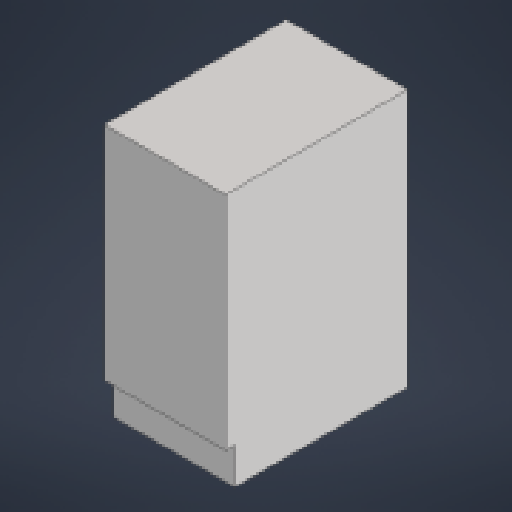
# Autodesk Inventor part: Mobile 40
Saved by Autodesk Inventor 2024.2 (Build 282272000, 272)
## iProperties
Created: 2025-08-13
Part Number: Mobile 40
Material: Generic
Document SubType Name: Modeling
Designer: Luca
Density: 1 g/cm^3
Appearance: Default
Author: Luca
Autodesk Inventor part; units mm, degrees
ref_plane "YZ Plane" through (0, 0, 0) normal (1, 0, 0) x (0, 1, 0)
ref_plane "XZ Plane" through (0, 0, 0) normal (0, 1, 0) x (-1, 0, 0)
ref_plane "XY Plane" through (0, 0, 0) normal (0, 0, 1) x (1, 0, 0)
sketch "Sketch1" plane through (0, 0, 0) normal (0, 1, 0) x (1, 0, 0)
  line L0 (200, 0) -> (-200, 0)
  line L1 (-200, 0) -> (-200, -600)
  line L2 (-200, -600) -> (200, -600)
  line L3 (200, -600) -> (200, 0)
  point P0 (0, 0)
  point P1 (0, 0)
  dimension "d0" = 400
  dimension "d1" = 600
  constraints: 8 end point, 2 parallel, 1 coincident, 1 horizontal, 1 midpoint, 1 perpendicular
  measures "d0" distance of L1.end L2.end
  measures "d1" distance of L0.end L1.end
extrude "Extrusion1" add sketch "Sketch1" along normal blind 850
sketch "Sketch2" plane through (-200, 0, 600) normal (0, 0, 1) x (-1, 0, 0)
  line L0 (-400, 0) -> (-400, -850) projected
  line L1 (0, 0) -> (0, -850) projected
  line L2 (-400, 0) -> (0, 0)
  line L3 (0, 0) -> (0, -120)
  line L4 (0, -120) -> (-400, -120)
  line L5 (-400, -120) -> (-400, 0)
  point P0 (-200, 0)
  point P1 (-400, -120)
  dimension "d4" = 120
  constraints: 8 end point, 2 parallel, 1 horizontal, 1 perpendicular, 1 point on line
  measures "d4" distance of L3.end L2.end
extrude "Extrusion2" cut sketch "Sketch2" against normal blind 30
body "Solid1"
